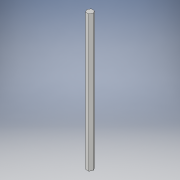
# Autodesk Inventor part: HexShaft12in
Saved by Autodesk Inventor 2018 (Build 220112000, 112)
## iProperties
Created: 2019-02-27
Part Number: HexShaft12in
Material: Generic
Document SubType Name: Modeling
Designer: snipe
Density: 1 g/cm^3
Appearance: Default
Author: snipe
Autodesk Inventor part; units mm, degrees
ref_plane "YZ Plane" through (0, 0, 0) normal (1, 0, 0) x (0, 1, 0)
ref_plane "XZ Plane" through (0, 0, 0) normal (0, 1, 0) x (-1, 0, 0)
ref_plane "XY Plane" through (0, 0, 0) normal (0, 0, 1) x (1, 0, 0)
sketch "Sketch1" plane through (0, 0, 0) normal (0, 1, 0) x (-1, 0, 0)
  line L0 (0, -8.89) -> (0, 8.89) projected
  line L1 (-10.2653, 0) -> (10.2653, 0) projected
  line L2 (10.2653, 0) -> (-10.2653, 0) projected
  line L3 (0, -8.89) -> (0, 8.89) projected
  line L4 (-7.3323, 0) -> (-3.6662, 6.35)
  line L5 (-3.6662, 6.35) -> (3.6662, 6.35)
  line L6 (3.6662, 6.35) -> (7.3323, 0)
  line L7 (7.3323, 0) -> (3.6662, -6.35)
  line L8 (3.6662, -6.35) -> (-3.6662, -6.35)
  line L9 (-3.6662, -6.35) -> (-7.3323, 0)
  point P0 (0, 0)
  point P1 (0, 0)
  dimension "d3" = 12.7
  constraints: 12 end point, 1 coincident, 1 point on line, 13 other
  measures "d3" distance between parallel lines of L5 L8
extrude "Extrusion1" add sketch "Sketch1" along normal mid plane 304.8
body "Solid1"
